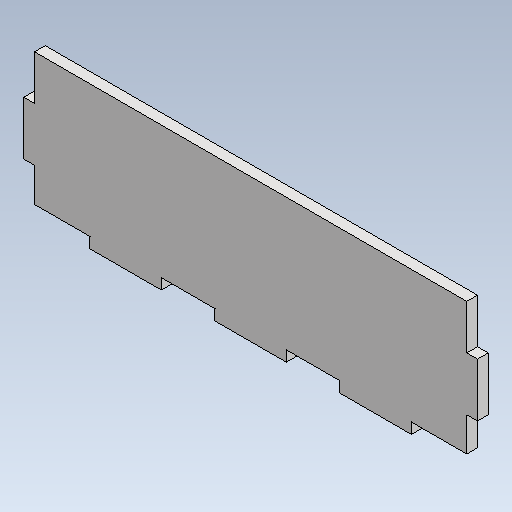
# Autodesk Inventor part: bed_acrylic_lower_front
Saved by Autodesk Inventor 2025 (Build 290162000, 162)
## iProperties
Created: 2025-08-24
Part Number: bed_acrylic_lower_front
Material: Generic
Document SubType Name: Modeling
Designer: HP
Density: 1 g/cm^3
Appearance: Default
Author: HP
Autodesk Inventor part; units mm, degrees
ref_plane "YZ Plane" through (0, 0, 0) normal (1, 0, 0) x (0, 1, 0)
ref_plane "XZ Plane" through (0, 0, 0) normal (0, 1, 0) x (-1, 0, 0)
ref_plane "XY Plane" through (0, 0, 0) normal (0, 0, 1) x (1, 0, 0)
sketch "Sketch1" plane through (0, 0, 0) normal (0, 0, 1) x (1, 0, 0)
  line L0 (-63.5, -20) -> (63.5, -20)
  line L1 (63.5, -20) -> (63.5, 20)
  line L2 (63.5, 20) -> (-63.5, 20)
  line L3 (-63.5, 20) -> (-63.5, -20)
  line L4 (-63.5, -20) -> (63.5, 20) construction
  line L5 (63.5, -20) -> (-63.5, 20) construction
  line L6 (-45, -17) -> (-25, -17) construction
  line L7 (-25, -17) -> (-25, -20)
  line L8 (-25, -20) -> (-45, -20)
  line L9 (-45, -20) -> (-45, -17)
  line L10 (-45, -17) -> (-25, -20) construction
  line L11 (-25, -17) -> (-45, -20) construction
  line L12 (-10, -17) -> (10, -17) construction
  line L13 (10, -17) -> (10, -20)
  line L14 (10, -20) -> (-10, -20)
  line L15 (-10, -20) -> (-10, -17)
  line L16 (-10, -17) -> (10, -20) construction
  line L17 (10, -17) -> (-10, -20) construction
  line L18 (25, -17) -> (45, -17) construction
  line L19 (45, -17) -> (45, -20)
  line L20 (45, -20) -> (25, -20)
  line L21 (25, -20) -> (25, -17)
  line L22 (25, -17) -> (45, -20) construction
  line L23 (45, -17) -> (25, -20) construction
  line L24 (-45, -17) -> (-63.5, -17)
  line L25 (-25, -17) -> (-10, -17)
  line L26 (10, -17) -> (25, -17)
  line L27 (45, -17) -> (63.5, -17)
  line L28 (-63.5, -7.5) -> (-60.5, -7.5)
  line L29 (-60.5, -7.5) -> (-60.5, 7.5) construction
  line L30 (-60.5, 7.5) -> (-63.5, 7.5)
  line L31 (-63.5, 7.5) -> (-63.5, -7.5)
  line L32 (-63.5, -7.5) -> (-60.5, 7.5) construction
  line L33 (-60.5, -7.5) -> (-63.5, 7.5) construction
  line L34 (-60.5, 7.5) -> (-60.5, 20)
  line L35 (-60.5, -7.5) -> (-60.5, -17)
  point P0 (0, 0)
  point P1 (-35, -18.5)
  point P2 (0, -18.5)
  point P3 (35, -18.5)
  point P4 (0, -20)
  point P5 (-62, 0)
  point P6 (-63.5, 0)
  point P7 (-63.5, -7.5)
  dimension "d0" = 127
  dimension "d1" = 40
  dimension "d2" = 20
  dimension "d3" = 3
  dimension "d4" = 20
  dimension "d5" = 3
  dimension "d6" = 20
  dimension "d7" = 3
  dimension "d8" = 35
  dimension "d9" = 35
  dimension "d10" = 15
  dimension "d11" = 3
  constraints: 72 end point, 12 midpoint, 10 parallel, 7 perpendicular, 5 horizontal, 5 point on line, 4 collinear, 1 horizontal alignment, 1 vertical, 1 vertical alignment
  measures "d0" distance between parallel lines of L1 L3
  measures "d1" distance between parallel lines of L0 L2
  measures "d2" distance of L7.end L8.end
  measures "d3" distance between parallel lines of L8 L6
  measures "d4" distance of L13.end L14.end
  measures "d5" distance between parallel lines of L14 L12
  measures "d6" distance of L19.end L20.end
  measures "d7" distance between parallel lines of L20 L18
  measures "d8" distance of point (0, -18.5) point (-35, -18.5)
  measures "d9" distance of point (35, -18.5) point (0, -18.5)
  measures "d10" distance between parallel lines of L28 L30
  measures "d11" distance between parallel lines of L31 L29
extrude "Extrusion1" add sketch "Sketch1" along normal blind 3 contours L9 L24 L35 L28 L3 L30 L34 L2 L1 L27 L19 L0 L21 L26 L13 L15 L25 L7 | L3 L28 L35 L24 | L3 L2 L34 L30
extrude "Extrusion2" cut sketch "Sketch1" along normal through all contours L3 L28 L35 L24 | L3 L2 L34 L30
mirror "Mirror1" about plane through (0, 0, 0) normal (1, 0, 0) of "Extrusion2"
equation "\"d4\" = d2"
equation "\"d5\" = d3"
equation "\"d6\" = d2"
equation "\"d7\" = d5"
equation "\"d9\" = d8"
equation "\"d11\" = d3"
body "Solid1"
